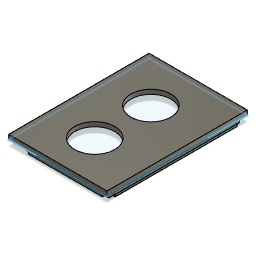
Buttons_Prototype (Autodesk Fusion 360 design; units mm, degrees)
Autodesk Fusion 360 part; units mm, degrees
(part 1 of 2)
sketch "Sketch1" plane through (0, 0, 0) normal (0, 0, 1) x (1, 0, 0)
  line L0 (-0.0637, 4.3306) -> (-17.0637, 4.3306)
  line L1 (-17.0637, 4.3306) -> (-17.0637, 0.3306)
  line L2 (-17.0637, 0.3306) -> (-0.0637, 0.3306)
  line L3 (-0.0637, 0.3306) -> (-0.0637, 4.3306)
  dimension "d1" = 17
  dimension "d13" = 4
  constraint horizontal L0
  constraint perpendicular L0 L1
  constraint horizontal L2
  constraint perpendicular L2 L3
  measures "d1" distance of L0.start L0.end
  measures "d13" distance of L0.start L2.end
extrude "Extrude1" add sketch "Sketch1" along normal blind 30 and the other way blind 30 makes body 1
mirror "Mirror1" about plane through (-0.0637, 0.3306, 0) normal (1, 0, 0) of bodies 1 makes body 2
combine "Combine1" operation add target body 2 tool bodies 1
sketch "Sketch2" plane through (0, 4.3306, 0) normal (0, 1, 0) x (-1, 0, 0)
  line L0 (-16.9363, 30) -> (-16.9363, -30)
  line L1 (-16.9363, -30) -> (17.0637, -30)
  line L2 (17.0637, -30) -> (17.0637, 30)
  line L3 (17.0637, 30) -> (-16.9363, 30)
  line L4 (-8.6363, -1.4) -> (-8.6363, 21)
  line L5 (-8.6363, 21) -> (8.7637, 21)
  line L6 (8.7637, 21) -> (8.7637, -1.4)
  line L7 (8.7637, -1.4) -> (-8.6363, -1.4)
  line L8 (17.0637, 22.0663) -> (-16.9363, 22.0663) construction
  line L9 (-16.3938, 30.8919) -> (16.5213, 30.8919) construction
  line L10 (0.0637, 30.8919) -> (0.0637, -2.5621) construction
  line L11 (-16.9363, 22.0663) -> (-16.9363, 33.4379) construction
  dimension "d43" = 17.4
  dimension "d44" = 22.4
  dimension "d45" = 17
  dimension "d46" = 8.7
  dimension "d47" = 9
  constraint vertical L4
  constraint horizontal L5
  constraint vertical L6
  constraint perpendicular L4 L7
  constraint coincident L2 L8.start
  constraint coincident L0 L8.end
  constraint perpendicular L0 L8
  constraint perpendicular L0 L9
  constraint midpoint L9 L10.start
  constraint perpendicular L9 L10
  constraint perpendicular L9 L11
  measures "d43" distance of L6.end L4.start
  measures "d44" distance of L6.end L5.end
  measures "d45" distance of L10 L11
  measures "d46" distance of L4 L10
  measures "d47" distance of L3 L5
extrude "Extrude2" cut sketch "Sketch2" against normal blind 10 contours L4 L5 L6 L7 bodies 2
sketch "Sketch4" plane through (0, 4.3306, 0) normal (0, 1, 0) x (-1, 0, 0)
  line L0 (-8.6363, 21) -> (8.7637, 21)
  line L1 (8.7637, 21) -> (8.7637, -1.4)
  line L2 (8.7637, -1.4) -> (-8.6363, -1.4)
  line L3 (-8.6363, -1.4) -> (-8.6363, 21)
  line L4 (-16.9363, 30) -> (-16.9363, -30)
  line L5 (-16.9363, -30) -> (17.0637, -30)
  line L6 (17.0637, -30) -> (17.0637, 30)
  line L7 (17.0637, 30) -> (-16.9363, 30)
  circle A0 centre (12.9637, 9.9412) radius 2.8284
  circle A1 centre (0.0637, -5.6) radius 2.8284
  circle A2 centre (-12.8363, 9.7728) radius 3.1
  circle A3 centre (0.0637, 25.2) radius 2.7801
  line L8 (0, 34) -> (-17, 34) construction
  line L9 (0, 34) -> (0, 33)
  line L10 (35.0061, 10.085) -> (-39.8532, 9.5965) construction
  line L11 (0.0637, -16.6918) -> (0.0637, 38.8918) construction
  dimension "d50" = 6.2
  dimension "d52" = 17
  dimension "d54" = 4.2
  dimension "d55" = 4.2
  dimension "d56" = 4.2
  dimension "d57" = 4.2
  dimension "d58" = 11.2
  dimension "d59" = 8.7
  constraint parallel L7 L8
  constraint perpendicular L8 L9
  constraint coincident A0.centre L10
  constraint coincident A2.centre L10
  constraint perpendicular L7 L11
  constraint coincident A1.centre L11
  constraint coincident A3.centre L11
  measures "d50" diameter of A2
  measures "d52" distance of L8.start L8.end
  measures "d54" distance of L3 A2.centre
  measures "d55" distance of L0 A3.centre
  measures "d56" distance of L1 A0.centre
  measures "d57" distance of L2 A1.centre
  measures "d58" distance of L2.end L10
  measures "d59" distance of L3 L11
extrude "Extrude3" cut sketch "Sketch4" against normal blind 1.7 contours A0 | A1 | A2 | A3 bodies 2
ref_plane "WorkPlane1" through (0, 0, 10) normal (0, 0, 1) x (1, 0, 0)
sketch "Sketch5" plane through (0, 0, 10) normal (0, 0, 1) x (1, 0, 0)
  line L0 (8.6363, 2.6306) -> (8.6363, 0.3626)
  line L1 (-8.7637, 0.3626) -> (-8.7637, 2.6306)
  line L2 (-8.7637, 2.6306) -> (-6.4957, 2.6306)
  line L3 (6.3683, 2.6306) -> (8.6363, 2.6306)
  line L4 (16.9363, 4.3306) -> (-17.0637, 4.3306)
  line L5 (-10, 0) -> (-8.8513, 0)
  line L6 (-8.7637, 2.6306) -> (8.6363, 2.6306) construction
  line L7 (-0.0637, -7.9052) -> (-0.0637, 9.0948) construction
  line L8 (16.9363, 4.3306) -> (16.9363, 0.3306)
  line L9 (-8.7637, 2.6306) -> (-6.4957, 2.6306)
  line L10 (-8.7637, 0.3626) -> (-6.4957, 2.6306)
  line L11 (-8.7637, 0.3626) -> (-5.573, 0.3626) construction
  line L12 (8.6363, 0.3626) -> (6.3683, 2.6306)
  line L13 (8.6363, 0.3626) -> (11.8101, 0.3626) construction
  dimension "d64" = 1.7
  dimension "d67" = 17.4
  dimension "d69" = 17
  dimension "d70" = 8.7
  dimension "d72" = 45
  dimension "d73" = 2.268
  dimension "d74" = 2.268
  dimension "d75" = 135
  constraint vertical L0
  constraint coincident L3.start L2
  constraint horizontal L5
  constraint vertical L7
  constraint horizontal L11
  constraint horizontal L13
  constraint perpendicular L0 L3
  constraint perpendicular L1 L6
  measures "d64" distance of L2 L4
  measures "d67" distance of L1.end L0.start
  measures "d69" distance of L7 L8
  measures "d70" distance of L0 L7
  measures "d72" angle of L10 L11
  measures "d73" distance of L0.start L3.start
  measures "d74" distance of L1.end L2.end
  measures "d75" angle of L12 L13
extrude "Extrude4" add sketch "Sketch5" along normal mid plane 10 bodies 2
extrude "Extrude5" add 1 faces at (-5.7304, 1.6639, 30) along direction (0, 0, 1) blind 39 on bodies 2 bodies 2
pattern_linear "R-Pattern1" count 1 spacing 0 along (-1, 0, 0) count 2 spacing 39 along (0, 0, 1) of "Extrude2", "Extrude3", "Extrude4"
extrude "Extrude6" cut 1 faces at (5.603, 1.6639, -30) along direction (0, 0, 1) blind 20 on bodies 2 bodies 2
sketch "Sketch1 (2)" plane through (0, 0, 0) normal (0, 1, 0) x (1, 0, 0) in component "Cap"
  line L0 (29.4953, 10.2833) -> (68.4953, 10.2833)
  line L1 (68.4953, 10.2833) -> (68.4953, -28.7167)
  line L2 (68.4953, -28.7167) -> (29.4953, -28.7167)
  line L3 (29.4953, -28.7167) -> (29.4953, 10.2833)
  dimension "d86" = 39
  dimension "d87" = 39
  constraint horizontal L0
  constraint vertical L1
  constraint horizontal L2
  constraint vertical L3
  measures "d86" distance of L0.start L0.end
  measures "d87" distance of L0.end L1.end
extrude "Extrude1'" add sketch "Sketch1 (2)" along normal blind 3 separate body makes body 3 in component "Cap"
sketch "Sketch2 (2)" plane through (0, 3, 0) normal (0, 1, 0) x (-1, 0, 0) in component "Cap"
  line L0 (-29.4953, 28.7167) -> (-68.4953, 28.7167)
  line L1 (-68.4953, 28.7167) -> (-68.4953, -10.2833)
  line L2 (-68.4953, -10.2833) -> (-29.4953, -10.2833)
  line L3 (-29.4953, -10.2833) -> (-29.4953, 28.7167)
  circle A0 centre (-48.9953, 9.2167) radius 14
  dimension "d90" = 28
  dimension "d114" = 19.5
  dimension "d115" = 19.5
  measures "d90" diameter of A0
  measures "d114" distance of L0 A0.centre
  measures "d115" distance of L1 A0.centre
extrude "Extrude2'" add sketch "Sketch2 (2)" along normal blind 12.9 contours A0 bodies 3 in component "Cap"
sketch "Sketch3" plane through (0, 0, 0) normal (0, -1, 0) x (1, 0, 0) in component "Cap"
  line L0 (-25.1467, 10) -> (-25.1467, -69)
  line L1 (-25.1467, -69) -> (-17.1467, -69)
  line L2 (-17.1467, -69) -> (-17.1467, 10)
  line L3 (68.4953, 28.7167) -> (29.4953, 28.7167)
  line L4 (29.4953, 28.7167) -> (29.4953, -10.2833)
  line L5 (29.4953, -10.2833) -> (68.4953, -10.2833)
  line L6 (68.4953, -10.2833) -> (68.4953, 28.7167)
  line L7 (48.9953, 40) -> (48.9953, -35.8515) construction
  line L8 (108.8863, 9.2167) -> (25.1963, 9.2167) construction
  line L9 (40.2953, 20.4167) -> (57.6953, 20.4167)
  line L10 (57.6953, 20.4167) -> (57.6953, -1.9833)
  line L11 (57.6953, -1.9833) -> (40.2953, -1.9833)
  line L12 (40.2953, -1.9833) -> (40.2953, 20.4167)
  circle A0 centre (36.0953, 9.2167) radius 3.1
  circle A1 centre (48.9953, 24.6167) radius 3.1
  circle A2 centre (61.8953, 9.2167) radius 3.1
  circle A3 centre (48.9953, -6.1833) radius 3.1
  dimension "d365" = 19.5
  dimension "d367" = 19.5
  dimension "d368" = 17.4
  dimension "d369" = 22.4
  dimension "d370" = 11.2
  dimension "d371" = 8.7
  dimension "d372" = 6.2
  dimension "d373" = 4.2
  dimension "d374" = 4.2
  dimension "d375" = 4.2
  dimension "d376" = 4.2
  constraint perpendicular L5 L7
  constraint perpendicular L6 L8
  constraint horizontal L9
  constraint vertical L10
  constraint horizontal L11
  constraint vertical L12
  constraint coincident L7 A1.centre
  constraint coincident L8 A2.centre
  constraint coincident L7 A3.centre
  constraint equal A1 A3
  constraint equal A2 A3
  constraint equal A0 A3
  constraint coincident L8 A0.centre
  measures "d365" distance of L3 L8
  measures "d367" distance of L6 L7
  measures "d368" distance of L9.start L9.end
  measures "d369" distance of L9.end L10.end
  measures "d370" distance of L8 L9
  measures "d371" distance of L7 L10
  measures "d372" diameter of A3
  measures "d373" distance of L12 A0.centre
  measures "d374" distance of L9 A1.centre
  measures "d375" distance of L11 A3.centre
  measures "d376" distance of L10 A2.centre
extrude "Extrude7" [suppressed]
extrude "Extrude3'" cut sketch "Sketch3" against normal blind 1.7 contours A0 | A1 | A2 | A3 bodies 3 in component "Cap"
sketch "Sketch5 (2)" plane through (0, 0, 0) normal (0, -1, 0) x (1, 0, 0) in component "Cap"
  line L0 (68.4953, 28.7167) -> (29.4953, 28.7167)
  line L1 (29.4953, 28.7167) -> (29.4953, -10.2833)
  line L2 (29.4953, -10.2833) -> (68.4953, -10.2833)
  line L3 (68.4953, -10.2833) -> (68.4953, 28.7167)
  line L4 (29.4953, 28.7167) -> (31.4953, 28.7167)
  line L5 (31.4953, 28.7167) -> (31.4953, -10.2833)
  line L6 (31.4953, -10.2833) -> (29.4953, -10.2833)
  line L7 (29.4953, -10.2833) -> (29.4953, 28.7167)
  line L8 (68.4953, -10.2833) -> (68.4953, 28.7167)
  circle A0 centre (48.9953, 24.6167) radius 3.1
  circle A1 centre (61.8953, 9.2167) radius 3.1
  circle A2 centre (36.0953, 9.2167) radius 3.1
  circle A3 centre (48.9953, -6.1833) radius 3.1
  line L9 (68.4953, 28.7167) -> (66.4953, 28.7167)
  line L10 (66.4953, 28.7167) -> (66.4953, -10.2833)
  line L11 (66.4953, -10.2833) -> (68.4953, -10.2833)
  line L12 (68.4953, -10.2833) -> (68.4953, 28.7167)
  dimension "d110" = 2
  dimension "d377" = 2
  constraint horizontal L4
  constraint vertical L5
  constraint horizontal L6
  constraint vertical L7
  constraint coincident L2 L5.end
  constraint coincident L0.end L1.start
  constraint vertical L8
  constraint coincident L0.start L3.end
  constraint horizontal L9
  constraint vertical L10
  constraint horizontal L11
  constraint vertical L12
  constraint coincident L2 L10.end
  measures "d110" distance of L0.end L4.end
  measures "d377" distance of L0.start L9.end
sketch "Sketch7" plane through (0, 0, 0) normal (0, 0, 1) x (1, 0, 0)
sketch "Sketch8" plane through (0, 4.3306, 0) normal (0, 1, 0) x (-1, 0, 0)
  line L0 (-16.9363, -10) -> (17.0637, -10)
  line L1 (17.0637, -10) -> (17.0637, 69)
  line L2 (17.0637, 69) -> (-16.9363, 69)
  line L3 (-16.9363, 69) -> (-16.9363, -10)
  line L4 (-8.6363, 21) -> (8.7637, 21)
  line L5 (8.7637, 21) -> (8.7637, -1.4)
  line L6 (8.7637, -1.4) -> (-8.6363, -1.4)
  line L7 (-8.6363, -1.4) -> (-8.6363, 21)
  circle A0 centre (12.9637, 9.9412) radius 2.8284
  circle A1 centre (0.0637, -5.6) radius 2.8284
  circle A2 centre (0.0637, 25.2) radius 2.7801
  circle A3 centre (-12.8363, 9.7728) radius 3.1
  line L8 (-8.6363, 60) -> (8.7637, 60)
  line L9 (8.7637, 60) -> (8.7637, 37.6)
  line L10 (8.7637, 37.6) -> (-8.6363, 37.6)
  line L11 (-8.6363, 37.6) -> (-8.6363, 60)
  circle A4 centre (12.9637, 48.9412) radius 2.8284
  circle A5 centre (0.0637, 33.4) radius 2.8284
  circle A6 centre (0.0637, 64.2) radius 2.7801
  circle A7 centre (-12.8363, 48.7728) radius 3.1
sketch "Sketch9" plane through (0, 3.3018, 0) normal (0, 1, 0) x (-1, 0, 0)
  line L0 (-24.8533, -10) -> (-16.8533, -10)
  line L1 (-16.8533, -10) -> (-16.8533, 69)
  line L2 (-16.8533, 69) -> (-24.8533, 69)
  line L3 (-24.8533, 69) -> (-24.8533, -10)
  circle A0 centre (-20.8533, 64) radius 1.4
  circle A1 centre (21.1467, 64) radius 1.4
  line L4 (17.1467, 69) -> (25.1467, 69)
  line L5 (25.1467, -10) -> (25.1467, 69)
  dimension "d116" = 2.8
  dimension "d117" = 5
  dimension "d118" = 5
  dimension "d119" = 4
  dimension "d120" = 4
  constraint equal A0 A1
  measures "d116" diameter of A0
  measures "d117" distance of L2 A0.centre
  measures "d118" distance of A1.centre L4
  measures "d119" distance of A1.centre L5
  measures "d120" distance of L3 A0.centre
extrude "Extrude8" cut sketch "Sketch9" against normal blind 4 contours A0 | A1 bodies 2
sketch "Sketch10" plane through (0, 3.3018, 0) normal (0, 1, 0) x (-1, 0, 0)
  circle A0 centre (-20.8533, 64) radius 1.4
  line L0 (-24.8533, -10) -> (-16.8533, -10)
  line L1 (-16.8533, -10) -> (-16.8533, 69)
  line L2 (-16.8533, 69) -> (-24.8533, 69)
  line L3 (-24.8533, 69) -> (-24.8533, -10)
  circle A1 centre (-20.8533, 64) radius 2.1574
  circle A2 centre (21.1467, 64) radius 2.1574
  circle A3 centre (21.1467, 64) radius 1.4
  dimension "d123" = 4.3148
  constraint concentric A0 A1
  constraint equal A1 A2
  constraint concentric A2 A3
  measures "d123" diameter of A1
extrude "Extrude9" cut sketch "Sketch10" against normal blind 1.2954 contours A1 | A2 bodies 2
pattern_linear "R-Pattern2" count 2 spacing 69 along (0, 0, -1) of "Extrude8", "Extrude9"
sketch "Sketch11" plane through (0, 3.3018, 0) normal (0, 1, 0) x (-1, 0, 0)
  circle A0 centre (-20.8533, -5) radius 2.1574
  circle A1 centre (-20.8533, 64) radius 2.1574
  line L0 (-24.8533, -10) -> (-16.8533, -10)
  line L1 (-16.8533, -10) -> (-16.8533, 69)
  line L2 (-16.8533, 69) -> (-24.8533, 69)
  line L3 (-16.8533, 0) -> (-24.8533, 0)
  line L4 (-24.8533, 0) -> (-24.8533, 59)
  line L5 (-24.8533, 59) -> (-16.8533, 59)
  line L6 (-16.8533, 59) -> (-16.8533, 0)
  line L7 (25.1467, 59) -> (17.1467, 59)
  line L8 (17.1467, 59) -> (17.1467, 0)
  line L9 (17.1467, 0) -> (25.1467, 0)
  line L10 (25.1467, 0) -> (25.1467, 59)
  line L11 (17.1467, 69) -> (25.1467, 69)
  line L12 (17.1467, -10) -> (25.1467, -10)
  line L13 (25.1467, -10) -> (25.1467, 69)
  dimension "d132" = 10
  dimension "d133" = 10
  dimension "d136" = 8
  dimension "d137" = 8
  dimension "d138" = 10
  dimension "d139" = 10
  constraint horizontal L3
  constraint vertical L4
  constraint horizontal L5
  constraint vertical L6
  constraint coincident L1 L3.start
  constraint vertical L8
  constraint horizontal L9
  constraint vertical L10
  constraint collinear L10 L13
  measures "d132" distance of L2 L5
  measures "d133" distance of L0 L3
  measures "d136" distance of L4.end L5.end
  measures "d137" distance of L7.start L7.end
  measures "d138" distance of L7 L11
  measures "d139" distance of L9 L12
extrude "Extrude10" cut sketch "Sketch11" against normal blind 4 contours L1 L3 L4 L5 L6 | L7 L8 L9 L10 L13 bodies 2
sketch "Sketch1 (3)" plane through (0, 0, 0) normal (0, 1, 0) x (1, 0, 0) in component "Cover top"
  circle A0 centre (116.6706, -10) radius 14.5
  line L0 (137.33, -17.9988) -> (133.9274, 3.8922)
  line L1 (133.9274, 3.8922) -> (113.268, 11.8909)
  line L2 (113.268, 11.8909) -> (96.0112, -2.0012)
  line L3 (96.0112, -2.0012) -> (99.4138, -23.8922)
  line L4 (99.4138, -23.8922) -> (120.0732, -31.8909)
  line L5 (120.0732, -31.8909) -> (137.33, -17.9988)
  point P0 (116.6706, -10)
  dimension "d140" = 29
  measures "d140" diameter of A0
extrude "Extrude1''" add sketch "Sketch1 (3)" along normal blind 3 separate body makes body 4 in component "Cover top"
fillet "Fillet1" radius 1 1 edges at (128.7016, 3, 24.9448) on bodies 4 in component "Cover top"
fillet "Fillet2" radius 1 9 edges at (109.2051, 3, 27.6831) (119.7578, 2.7071, 31.7688) (120.0732, 1, 31.8909) (137.33, 1, 17.9988) (137.2781, 2.7071, 17.6646) (135.54, 3, 6.4828) (123.5977, 3, -7.8916) (97.7125, 3, 12.9467) (104.6396, 3, -4.9448) on bodies 4 in component "Cover top"
sketch "Sketch15" plane through (0, 0, 0) normal (0, 1, 0) x (-1, 0, 0)
sketch "Sketch1 (4)" plane through (0, 0, 0) normal (0, 0, 1) x (1, 0, 0) in component "Box"
  line L0 (-116.6556, 53.5174) -> (-46.6556, 53.5174)
  line L1 (-46.6556, 53.5174) -> (-46.6556, -6.4826)
  line L2 (-46.6556, -6.4826) -> (-116.6556, -6.4826)
  line L3 (-116.6556, -6.4826) -> (-116.6556, 53.5174)
  dimension "d149" = 70
  dimension "d150" = 60
  constraint horizontal L0
  constraint vertical L1
  constraint horizontal L2
  constraint vertical L3
  measures "d149" distance of L0.start L0.end
  measures "d150" distance of L0.start L2.end
extrude "Extrude1'''" add sketch "Sketch1 (4)" along normal blind 50 and the other way blind 50 separate body makes body 5 in component "Box"
sketch "Sketch2 (3)" plane through (-93.9993, 53.5174, 74.8295) normal (0, 1, 0) x (-1, 0, 0) in component "Box"
  line L0 (22.6563, -124.8295) -> (22.6563, -24.8295)
  line L1 (22.6563, -24.8295) -> (-47.3437, -24.8295)
  line L2 (-47.3437, -24.8295) -> (-47.3437, -124.8295)
  line L3 (-47.3437, -124.8295) -> (22.6563, -124.8295)
  line L4 (2.6563, -114.8295) -> (-27.3437, -114.8295)
  line L5 (-27.3437, -114.8295) -> (-27.3437, -34.8295)
  line L6 (-27.3437, -34.8295) -> (2.6563, -34.8295)
  line L7 (2.6563, -34.8295) -> (2.6563, -114.8295)
  line L8 (-11.4915, -124.8295) -> (-11.4915, -24.8295) construction
  dimension "d155" = 20
  dimension "d156" = 20
  dimension "d157" = 10
  dimension "d158" = 10
  constraint horizontal L4
  constraint vertical L5
  constraint horizontal L6
  constraint vertical L7
  constraint coincident L3 L8.start
  constraint coincident L1 L8.end
  constraint perpendicular L1 L8
  measures "d155" distance of L0 L7
  measures "d156" distance of L2 L5
  measures "d157" distance of L3 L4
  measures "d158" distance of L1 L6
sketch "Sketch4 (2)" plane through (0, 53.5174, 0) normal (0, 1, 0) x (-1, 0, 0) in component "Box"
  line L0 (66.6556, -40) -> (66.6556, 40)
  line L1 (66.6556, 40) -> (96.6556, 40)
  line L2 (96.6556, 40) -> (96.6556, -40)
  line L3 (96.6556, -40) -> (66.6556, -40)
  line L4 (116.6556, -50) -> (116.6556, 50)
  line L5 (116.6556, 50) -> (46.6556, 50)
  line L6 (46.6556, -50) -> (116.6556, -50)
  line L7 (113.6556, -47) -> (49.6556, -47)
  line L8 (49.6556, 47) -> (113.6556, 47)
  line L9 (113.6556, 47) -> (113.6556, -47)
  line L10 (116.6556, -50) -> (116.6556, 50)
  line L11 (116.6556, 50) -> (46.6556, 50)
  line L12 (46.6556, 50) -> (46.6556, -50)
  line L13 (46.6556, -50) -> (116.6556, -50)
  line L14 (49.6556, 47) -> (49.6556, 40)
  line L15 (49.6556, 40) -> (49.6556, -47)
  dimension "d167" = 3
  dimension "d170" = 3
  dimension "d171" = 3
  dimension "d260" = 3
  constraint horizontal L7
  constraint horizontal L8
  constraint vertical L9
  constraint perpendicular L8 L14
  constraint coincident L7 L15.end
  constraint perpendicular L7 L15
  measures "d167" distance of L4 L9
  measures "d170" distance of L5 L8
  measures "d171" distance of L6 L7
  measures "d260" distance of L12 L15
extrude "Extrude3''" cut sketch "Sketch4 (2)" against normal blind 23 contours L7 L8 L9 L14 L15 bodies 5 in component "Box"
sketch "Sketch6" plane through (0, 0, 0) normal (0, 1, 0) x (1, 0, 0) in component "Box"
sketch "Sketch7 (2)" plane through (0, 30.5174, 0) normal (0, 1, 0) x (-1, 0, 0) in component "Box"
  line L0 (42.6223, -47) -> (98.8748, -47) construction
  line L1 (110.5382, -35) -> (59.6556, -35) construction
  line L2 (53.4031, 35) -> (110.5382, 35) construction
  line L3 (15.5936, 0) -> (180.7808, 0) construction
  line L4 (105.8748, -50) -> (35.8748, -50)
  circle A0 centre (102.6556, -30) radius 1.4
  circle A1 centre (60.6556, -30) radius 1.4
  circle A2 centre (60.6556, 30) radius 1.4
  circle A3 centre (102.6556, 30) radius 1.4
  line L5 (106.6556, -35) -> (56.6556, -35)
  line L6 (56.6556, -35) -> (56.6556, 35)
  line L7 (56.6556, 35) -> (106.6556, 35)
  line L8 (106.6556, 35) -> (106.6556, -35)
  line L9 (124.5176, 0) -> (30.7808, 0) construction
  line L10 (81.6556, 61.2819) -> (81.6556, -48.7181) construction
  line L11 (116.6556, -50) -> (116.6556, 50)
  line L12 (98.6556, -35) -> (64.6556, -35)
  line L13 (64.6556, -35) -> (64.6556, 35) construction
  line L14 (64.6556, 35) -> (98.6556, 35)
  line L15 (98.6556, 35) -> (98.6556, -35) construction
  line L16 (49.6556, -47) -> (113.6556, -47)
  line L17 (113.6556, -47) -> (113.6556, 47)
  line L18 (113.6556, 47) -> (49.6556, 47)
  line L19 (49.6556, 47) -> (49.6556, -47)
  line L20 (96.6556, 40) -> (96.6556, -40)
  line L21 (96.6556, -40) -> (66.6556, -40)
  line L22 (66.6556, -40) -> (66.6556, 40)
  line L23 (66.6556, 40) -> (96.6556, 40)
  dimension "d193" = 70
  dimension "d194" = 50
  dimension "d195" = 35
  dimension "d196" = 2.8
  dimension "d197" = 2.8
  dimension "d198" = 5
  dimension "d199" = 5
  dimension "d215" = 50
  dimension "d216" = 35
  dimension "d217" = 25
  dimension "d218" = 70
  dimension "d219" = 35
  dimension "d220" = 8
  dimension "d221" = 8
  dimension "d222" = 4
  dimension "d223" = 5
  dimension "d224" = 5
  dimension "d225" = 4
  dimension "d226" = 4
  dimension "d227" = 5
  dimension "d228" = 4
  constraint horizontal L1
  constraint horizontal L2
  constraint horizontal L3
  constraint equal A0 A1
  constraint equal A1 A2
  constraint horizontal L5
  constraint vertical L6
  constraint horizontal L7
  constraint vertical L8
  constraint coincident L3 L9.start
  constraint coincident L3 L9.end
  constraint perpendicular L8 L9
  constraint perpendicular L4 L10
  constraint horizontal L12
  constraint vertical L13
  constraint horizontal L14
  constraint vertical L15
  constraint coincident L2 L13.end
  constraint coincident L5 L12.start
  measures "d193" distance of L1.start L2.end
  measures "d194" distance of L3 L4
  measures "d195" distance of L2 L3
  measures "d196" diameter of A3
  measures "d197" diameter of A0
  measures "d198" distance of L2 A2.centre
  measures "d199" distance of L2 A3.centre
  measures "d215" distance of L5.start L5.end
  measures "d216" distance of L10 L11
  measures "d217" distance of L8 L10
  measures "d218" distance of L5.end L6.end
  measures "d219" distance of L3 L5
  measures "d220" distance of L8 L15
  measures "d221" distance of L6 L13
  measures "d222" distance of A1.centre L13
  measures "d223" distance of A1.centre L5
  measures "d224" distance of L1 A0.centre
  measures "d225" distance of A0.centre L8
  measures "d226" distance of A3.centre L15
  measures "d227" distance of A3.centre L7
  measures "d228" distance of A2.centre L13
sketch "Sketch18" plane through (0, 0, 0) normal (0, 1, 0) x (1, 0, 0)
sketch "Sketch1 (5)" plane through (0, 0, 0) normal (0, 1, 0) x (1, 0, 0) in component "Cover"
  line L0 (-40.9344, -0.0564) -> (29.0656, -0.0564)
  line L1 (29.0656, -0.0564) -> (29.0656, -100.0564)
  line L2 (29.0656, -100.0564) -> (-40.9344, -100.0564)
  line L3 (-40.9344, -100.0564) -> (-40.9344, -0.0564)
  dimension "d240" = 70
  dimension "d241" = 100
  constraint horizontal L0
  constraint vertical L1
  constraint horizontal L2
  constraint vertical L3
  measures "d240" distance of L0.start L0.end
  measures "d241" distance of L0.end L1.end
extrude "Extrude1''''" add sketch "Sketch1 (5)" along normal blind 3.175 separate body makes body 6 in component "Cover"
sketch "Sketch2 (4)" plane through (0, 3.175, 0) normal (0, 1, 0) x (-1, 0, 0) in component "Cover"
  line L0 (40.9344, 100.0564) -> (-29.0656, 100.0564)
  line L1 (-29.0656, 100.0564) -> (-29.0656, 0.0564)
  line L2 (-29.0656, 0.0564) -> (40.9344, 0.0564)
  line L3 (40.9344, 0.0564) -> (40.9344, 100.0564)
  line L4 (23.3344, 8.9564) -> (-15.6656, 8.9564)
  line L5 (-15.6656, 8.9564) -> (-15.6656, 87.9564)
  line L6 (-15.6656, 87.9564) -> (23.3344, 87.9564)
  line L7 (23.3344, 87.9564) -> (23.3344, 8.9564)
  line L8 (3.8344, 0.0564) -> (3.8344, 130.0564) construction
  line L9 (-78.285, 47.9564) -> (126.7344, 47.9564) construction
  line L10 (-29.0656, 0.0564) -> (-29.0656, 100.0564) construction
  line L11 (40.9344, 0.0564) -> (-29.0656, 0.0564) construction
  circle A0 centre (3.8344, 28.4564) radius 14.25
  line L12 (21.4134, 8.9564) -> (21.4134, 47.9564) construction
  circle A1 centre (3.8344, 68.4564) radius 14.25
  line L13 (23.3344, 48.9564) -> (-98.2656, 48.9564) construction
  dimension "d247" = 39
  dimension "d248" = 79
  dimension "d249" = 32.9
  dimension "d250" = 47.9
  dimension "d251" = 39
  dimension "d253" = 28.5
  dimension "d254" = 19.5
  dimension "d255" = 39
  dimension "d256" = 19.5
  dimension "d257" = 19.5
  constraint horizontal L4
  constraint vertical L5
  constraint horizontal L6
  constraint vertical L7
  constraint coincident L2 L8.start
  constraint perpendicular L0 L8
  constraint perpendicular L3 L9
  constraint coincident L8 A0.centre
  constraint coincident L4 L12.start
  constraint coincident L9 L12.end
  constraint perpendicular L9 L12
  constraint coincident L8 A1.centre
  constraint equal A0 A1
  constraint coincident L7 L13.start
  constraint perpendicular L7 L13
  measures "d247" distance of L4.start L4.end
  measures "d248" distance of L4.start L6.end
  measures "d249" distance of L8 L10
  measures "d250" distance of L9 L11
  measures "d251" distance of L4 L9
  measures "d253" diameter of A0
  measures "d254" distance of L9 A0.centre
  measures "d255" distance of L6 L13
  measures "d256" distance of L6 A1.centre
  measures "d257" distance of L5 L8
extrude "Extrude2''" cut sketch "Sketch2 (4)" against normal blind 20 contours A0 | A1 bodies 6 in component "Cover"
sketch "Sketch9 (2)" plane through (0, 53.5174, 0) normal (0, 1, 0) x (-1, 0, 0) in component "Box"
  line L0 (49.6556, 47) -> (113.6556, 47)
  line L1 (113.6556, 47) -> (113.6556, -47)
  line L2 (113.6556, -47) -> (49.6556, -47)
  line L3 (46.6556, 50) -> (46.6556, -50)
  line L4 (46.6556, -50) -> (116.6556, -50)
  line L5 (116.6556, -50) -> (116.6556, 50)
  line L6 (116.6556, 50) -> (46.6556, 50)
  line L7 (49.6556, -47) -> (49.6556, 47)
sketch "Sketch10 (2)" plane through (0, 53.5174, 0) normal (0, 1, 0) x (-1, 0, 0) in component "Box"
sketch "Sketch11 (2)" plane through (-81.6556, 53.5174, 0) normal (0, 1, 0) x (-1, 0, 0) in component "Box"
ref_plane "WorkPlane2" through (-81.6556, 23.5174, 30) normal (0, 0, 1) x (1, 0, 0) in component "Box"
sketch "Sketch8 (2)" plane through (0, 0, 50) normal (0, 0, 1) x (1, 0, 0) in component "Box"
  line L0 (-116.6556, -6.4826) -> (-46.6556, -6.4826)
  line L1 (-46.6556, -6.4826) -> (-46.6556, 53.5174)
  line L2 (-46.6556, 53.5174) -> (-116.6556, 53.5174)
  line L3 (-116.6556, 53.5174) -> (-116.6556, -6.4826)
  line L4 (-111.6556, -3.4826) -> (-51.6556, -3.4826)
  line L5 (-51.6556, -3.4826) -> (-51.6556, 21.5174)
  line L6 (-51.6556, 21.5174) -> (-111.6556, 21.5174)
  line L7 (-111.6556, 21.5174) -> (-111.6556, -3.4826)
  dimension "d232" = 60
  dimension "d233" = 3
  dimension "d234" = 25
  dimension "d235" = 5
  constraint horizontal L4
  constraint vertical L5
  constraint horizontal L6
  constraint vertical L7
  measures "d232" distance of L4.start L4.end
  measures "d233" distance of L0 L4
  measures "d234" distance of L4.start L6.end
  measures "d235" distance of L3 L7
extrude "Extrude6'" cut sketch "Sketch8 (2)" along normal blind -5 and the other way blind 95 contours L4 L5 L6 L7 bodies 5 in component "Box"
sketch "Sketch17" plane through (-43.9231, 0, 0) normal (1, 0, 0) x (0, 0, -1)
  line L0 (22.0668, 15.9767) -> (-71.9332, 15.9767)
  line L1 (-71.9332, 15.9767) -> (-71.9332, -7.0233)
  line L2 (-71.9332, -7.0233) -> (22.0668, -7.0233)
  line L3 (22.0668, -7.0233) -> (22.0668, 15.9767)
extrude "Extrude5'" cut sketch "Sketch7 (2)" against normal blind 10 contours A0 | A1 | A2 | A3 bodies 5 in component "Box"
sketch "Sketch14" plane through (0, 0, 50) normal (0, 0, 1) x (1, 0, 0) in component "Box"
  line L0 (-116.6556, -6.4826) -> (-46.6556, -6.4826)
  line L1 (-46.6556, -6.4826) -> (-46.6556, 53.5174)
  line L2 (-46.6556, 53.5174) -> (-116.6556, 53.5174)
  line L3 (-116.6556, 53.5174) -> (-116.6556, -6.4826)
  line L4 (-48.6556, 51.5174) -> (-114.6556, 51.5174)
  line L5 (-114.6556, 51.5174) -> (-114.6556, 49.5174)
  line L6 (-114.6556, 49.5174) -> (-48.6556, 49.5174)
  line L7 (-116.6556, 53.5174) -> (-46.6556, 53.5174)
  line L8 (-48.6556, 51.5174) -> (-48.6556, 49.5174)
  line L9 (-46.6556, 53.5174) -> (-46.6556, -6.4826)
  dimension "d263" = 2
  dimension "d264" = 2
  dimension "d265" = 2
  dimension "d337" = 2
  constraint horizontal L4
  constraint vertical L5
  constraint horizontal L6
  constraint perpendicular L6 L8
  measures "d263" distance of L4 L7
  measures "d264" distance of L4.start L6.end
  measures "d265" distance of L3 L5
  measures "d337" distance of L8 L9
extrude "Extrude8'" cut sketch "Sketch14" against normal blind 3 from surface at -2 contours L4 L5 L6 L8 bodies 5 in component "Box"
sketch "Sketch15 (2)" plane through (-46.6556, 0, 0) normal (1, 0, 0) x (0, 0, 1) in component "Box"
  line L0 (-50, -6.4826) -> (50, -6.4826)
  line L1 (-48, 51.5174) -> (-48, 49.1197)
  line L2 (46, 49.1197) -> (46, 51.5174)
  line L3 (-50, -53.5174) -> (50, -53.5174)
  line L4 (50, -53.5174) -> (50, 6.4826)
  line L5 (50, 6.4826) -> (-50, 6.4826)
  line L6 (-50, 6.4826) -> (-50, -53.5174)
  constraint vertical L1
  constraint vertical L2
sketch "Sketch16" plane through (-46.6556, 0, 0) normal (1, 0, 0) x (0, 0, 1) in component "Box"
  line L0 (48, -51.5174) -> (-48, -51.5174)
  line L1 (-48, -51.5174) -> (-48, -49.5174)
  line L2 (-48, -49.5174) -> (48, -49.5174)
  line L3 (48, -49.5174) -> (48, -51.5174)
  line L4 (-50, -53.5174) -> (50, -53.5174)
  line L5 (-50, 6.4826) -> (-50, -53.5174)
  line L6 (50, -53.5174) -> (50, 6.4826)
  dimension "d274" = 2
  dimension "d275" = 2
  dimension "d276" = 2
  dimension "d280" = 2
  constraint horizontal L0
  constraint vertical L1
  constraint horizontal L2
  constraint vertical L3
  measures "d274" distance of L0 L4
  measures "d275" distance of L1 L5
  measures "d276" distance of L2.end L6
  measures "d280" distance of L0.end L1.end
extrude "Extrude9'" cut sketch "Sketch16" against normal blind 3 from surface at -2 bodies 5 in component "Box"
sketch "Sketch17 (2)" plane through (0, 0, -50) normal (0, 0, -1) x (-1, 0, 0) in component "Box"
  line L0 (46.6556, -6.4826) -> (116.6556, -6.4826)
  line L1 (116.6556, -6.4826) -> (116.6556, 53.5174)
  line L2 (116.6556, 53.5174) -> (46.6556, 53.5174)
  line L3 (46.6556, 53.5174) -> (46.6556, -6.4826)
  line L4 (114.6556, 51.5174) -> (48.6556, 51.5174)
  line L5 (48.6556, 51.5174) -> (48.6556, 49.5174)
  line L6 (48.6556, 49.5174) -> (114.6556, 49.5174)
  line L7 (114.6556, 49.5174) -> (114.6556, 51.5174)
  dimension "d281" = 2
  dimension "d282" = 2
  dimension "d283" = 2
  dimension "d284" = 2
  constraint horizontal L4
  constraint vertical L5
  constraint horizontal L6
  constraint vertical L7
  measures "d281" distance of L4.start L6.end
  measures "d282" distance of L2 L4
  measures "d283" distance of L1 L7
  measures "d284" distance of L3 L5
sketch "Sketch18 (2)" plane through (-116.6556, 0, 0) normal (-1, 0, 0) x (0, 0, 1) in component "Box"
  line L0 (-50, -6.4826) -> (50, -6.4826)
  line L1 (50, -6.4826) -> (50, 53.5174)
  line L2 (50, 53.5174) -> (-50, 53.5174)
  line L3 (-50, 53.5174) -> (-50, -6.4826)
  line L4 (-47, -1.4826) -> (47, -1.4826)
  line L5 (47, -1.4826) -> (47, 53.5174)
  line L6 (47, 53.5174) -> (-47, 53.5174)
  line L7 (-47, 53.5174) -> (-47, -1.4826)
  dimension "d285" = 3
  dimension "d286" = 5
  dimension "d287" = 3
  constraint horizontal L4
  constraint vertical L5
  constraint horizontal L6
  constraint vertical L7
  constraint coincident L2 L5.end
  measures "d285" distance of L1 L5
  measures "d286" distance of L0 L4
  measures "d287" distance of L3 L7
extrude "Extrude10'" cut sketch "Sketch18 (2)" against normal blind 5 contours L2 L4 L5 L6 L7 bodies 5 in component "Box"
sketch "Sketch19" plane through (0, 0, 47) normal (0, 0, -1) x (-1, 0, 0) in component "Box"
  line L0 (114.6556, 49.5174) -> (49.6556, 49.5174)
  line L1 (111.6556, 30.5174) -> (111.6556, -1.4826)
  line L2 (111.6556, -1.4826) -> (116.6556, -1.4826)
  line L3 (116.6556, -1.4826) -> (116.6556, 53.5174)
  line L4 (116.6556, 53.5174) -> (49.6556, 53.5174)
  line L5 (49.6556, 51.5174) -> (114.6556, 51.5174)
  line L6 (114.6556, 51.5174) -> (114.6556, 49.5174)
  line L7 (114.6556, 53.467) -> (112.6556, 53.467)
  line L8 (112.6556, 53.467) -> (112.6556, -1.4826)
  line L9 (112.6556, -1.4826) -> (114.6556, -1.4826)
  line L10 (114.6556, -1.4826) -> (114.6556, 53.467)
  line L11 (116.6556, -6.4826) -> (116.6556, 53.5174)
  line L12 (46.6556, -6.4826) -> (116.6556, -6.4826)
  line L13 (49.6556, 53.5174) -> (49.6556, 51.5174)
  line L14 (49.6556, 49.5174) -> (49.6556, 30.5174)
  line L15 (49.6556, 30.5174) -> (111.6556, 30.5174)
  line L16 (114.6556, 53.467) -> (114.6556, 49)
  dimension "d290" = 2
  dimension "d293" = 5
  dimension "d294" = 2
  constraint vertical L8
  constraint horizontal L9
  constraint vertical L10
  constraint coincident L10 L16.end
  constraint perpendicular L0 L16
  measures "d290" distance of L10 L11
  measures "d293" distance of L9 L12
  measures "d294" distance of L8.end L9.end
extrude "Extrude11" cut sketch "Sketch19" against normal blind 2 contours L0 L2 L8 L9 L10 L16 | L0 L5 L6 L8 L10 L16 | L5 L7 L8 L10 L16 bodies 5 in component "Box"
sketch "Sketch4 (3)" plane through (0, 0, 0) normal (0, 1, 0) x (1, 0, 0) in component "Cover"
  line L0 (20.0656, -96.5564) -> (-38.7344, -96.5564)
  line L1 (-38.7344, -96.5564) -> (-38.7344, -3.5564)
  line L2 (-38.7344, -3.5564) -> (20.0656, -3.5564)
  line L3 (20.0656, -6.5564) -> (-35.7344, -6.5564)
  line L4 (-35.7344, -6.5564) -> (-35.7344, -93.5564)
  line L5 (-35.7344, -93.5564) -> (20.0656, -93.5564)
  line L6 (20.0656, -96.5564) -> (20.0656, -93.5564)
  line L7 (29.0656, -0.0564) -> (29.0656, -100.0564)
  line L8 (29.0656, -100.0564) -> (-40.9344, -100.0564)
  line L9 (-40.9344, -100.0564) -> (-40.9344, -0.0564)
  line L10 (-40.9344, -0.0564) -> (29.0656, -0.0564)
  line L11 (20.0656, -6.5564) -> (20.0656, -3.5564)
  dimension "d308" = 3.5
  dimension "d311" = 3
  dimension "d312" = 3.5
  dimension "d320" = 3
  dimension "d338" = 9
  dimension "d385" = 58.8
  dimension "d386" = 55.8
  dimension "d387" = 9
  constraint horizontal L0
  constraint perpendicular L0 L1
  constraint perpendicular L1 L2
  constraint perpendicular L3 L4
  constraint perpendicular L5 L6
  constraint coincident L5 L6.end
  constraint perpendicular L3 L11
  measures "d308" distance of L0 L8
  measures "d311" distance of L0.start L5.end
  measures "d312" distance of L2 L10
  measures "d320" distance of L1 L4
  measures "d338" distance of L7 L11
  measures "d385" distance of L0.start L0.end
  measures "d386" distance of L4.end L5.end
  measures "d387" distance of L6 L7
extrude "Extrude3'''" add sketch "Sketch4 (3)" against normal blind 4 contours L0 L1 L2 L3 L4 L5 L6 L11 bodies 6 in component "Cover"
sketch "Sketch5 (3)" plane through (0, 0, 96.5564) normal (0, 0, 1) x (1, 0, 0) in component "Cover"
  line L0 (20.0656, 0) -> (-38.7344, 0)
  line L1 (-38.7344, 0) -> (-38.7344, -4)
  line L2 (-38.7344, -4) -> (20.0656, -4)
  line L3 (20.0656, -4) -> (20.0656, 0)
  line L4 (-35.7344, -2.5) -> (17.0656, -2.5)
  line L5 (17.0656, -2.5) -> (17.0656, -4)
  line L6 (17.0656, -4) -> (-35.7344, -4)
  line L7 (-35.7344, -4) -> (-35.7344, -2.5)
  line L8 (29.0656, 0) -> (-40.9344, 0)
  dimension "d321" = 2.5
  dimension "d322" = 1.5
  dimension "d323" = 3
  dimension "d324" = 3
  constraint horizontal L4
  constraint vertical L5
  constraint horizontal L6
  constraint vertical L7
  measures "d321" distance of L4 L8
  measures "d322" distance of L4.end L5.end
  measures "d323" distance of L1 L7
  measures "d324" distance of L3 L5
extrude "Extrude4'" add sketch "Sketch5 (3)" along normal blind 1.5 contours L2 L4 L5 L6 L7 bodies 6 in component "Cover"
sketch "Sketch6 (2)" plane through (0, 0, 3.5564) normal (0, 0, -1) x (-1, 0, 0) in component "Cover"
  line L0 (38.7344, 0) -> (-20.0656, 0)
  line L1 (-20.0656, -4) -> (38.7344, -4)
  line L2 (38.7344, -4) -> (38.7344, 0)
  line L3 (-17.0656, -2.5) -> (35.7344, -2.5)
  line L4 (35.7344, -2.5) -> (35.7344, -4)
  line L5 (35.7344, -4) -> (-17.0656, -4)
  line L6 (-17.0656, -4) -> (-17.0656, -2.5)
  line L7 (40.9344, 0) -> (-29.0656, 0)
  line L8 (-20.0656, 0) -> (-20.0656, -4)
  dimension "d327" = 2.5
  dimension "d328" = 3
  constraint horizontal L3
  constraint vertical L4
  constraint horizontal L5
  constraint vertical L6
  constraint coincident L1 L4.end
  measures "d327" distance of L3 L7
  measures "d328" distance of L2 L4
extrude "Extrude5''" add sketch "Sketch6 (2)" along normal blind 1.5 contours L1 L3 L4 L5 L6 bodies 6 in component "Cover"
sketch "Sketch7 (3)" plane through (-38.7344, 0, 0) normal (-1, 0, 0) x (0, 0, 1) in component "Cover"
  line L0 (96.5564, 0) -> (3.5564, 0)
  line L1 (3.5564, 0) -> (3.5564, -4)
  line L2 (3.5564, -4) -> (96.5564, -4)
  line L3 (96.5564, -4) -> (96.5564, 0)
  line L4 (6.5564, -2.5) -> (93.5564, -2.5)
  line L5 (93.5564, -2.5) -> (93.5564, -4)
  line L6 (93.5564, -4) -> (6.5564, -4)
  line L7 (6.5564, -4) -> (6.5564, -2.5)
  line L8 (100.0564, 0) -> (0.0564, 0)
  dimension "d332" = 2.5
  dimension "d333" = 3
  dimension "d334" = 3
  constraint horizontal L4
  constraint vertical L5
  constraint horizontal L6
  constraint vertical L7
  constraint coincident L2 L5.end
  measures "d332" distance of L4 L8
  measures "d333" distance of L3 L5
  measures "d334" distance of L1 L7
extrude "Extrude6''" add sketch "Sketch7 (3)" along normal blind 1.5 contours L2 L4 L5 L6 L7 bodies 6 in component "Cover"
sketch "Sketch20" plane through (-111.6556, 0, 0) normal (-1, 0, 0) x (0, 0, 1) in component "Box"
  line L0 (45, 21.5174) -> (45, -1.4826)
  line L1 (45, -1.4826) -> (47, -1.4826)
  line L2 (47, -1.4826) -> (47, 30.5174)
  line L3 (47, 30.5174) -> (-47, 30.5174)
  line L4 (-47, 30.5174) -> (-47, -1.4826)
  line L5 (-47, -1.4826) -> (-45, -1.4826)
  line L6 (-45, -1.4826) -> (-45, 21.5174)
  line L7 (-45, 21.5174) -> (45, 21.5174)
sketch "Sketch8 (3)" plane through (0, 0, 0) normal (0, 1, 0) x (1, 0, 0) in component "Cover"
sketch "Sketch21" plane through (-93.9993, 53.5174, 74.8295) normal (0, 1, 0) x (-1, 0, 0) in component "Box"
  line L0 (22.6563, -124.8295) -> (22.6563, -24.8295)
  line L1 (20.6563, -27.8372) -> (18.6563, -27.8372)
  line L2 (18.6563, -27.8372) -> (18.6563, -25.9523)
  line L3 (18.6563, -25.9523) -> (20.6563, -25.9523)
  line L4 (20.6563, -25.9523) -> (20.6563, -27.8372)
  dimension "d344" = 2
  dimension "d345" = 2
  constraint horizontal L1
  constraint vertical L2
  constraint horizontal L3
  constraint vertical L4
  measures "d344" distance of L2.end L3.end
  measures "d345" distance of L0 L4
extrude "Extrude12" cut sketch "Sketch21" against normal blind 1 bodies 5 in component "Box"
sketch "Sketch22" plane through (0, 0, -47) normal (0, 0, 1) x (1, 0, 0) in component "Box"
  line L0 (-111.6556, 30.5174) -> (-49.6556, 30.5174)
  line L1 (-49.6556, 30.5174) -> (-49.6556, 49.5174)
  line L2 (-49.6556, 49.5174) -> (-51.6556, 49.5174)
  line L3 (-51.6556, 49.5174) -> (-51.6556, 51.5174)
  line L4 (-51.6556, 51.5174) -> (-49.6556, 51.5174)
  line L5 (-49.6556, 51.5174) -> (-49.6556, 53.5174)
  line L6 (-49.6556, 53.5174) -> (-116.6556, 53.5174)
  line L7 (-116.6556, 53.5174) -> (-116.6556, -1.4826)
  line L8 (-116.6556, -1.4826) -> (-111.6556, -1.4826)
  line L9 (-111.6556, -1.4826) -> (-111.6556, 30.5174)
  line L10 (-114.6556, -1.4826) -> (-112.6556, -1.4826)
  line L11 (-112.1556, -1.4826) -> (-112.1556, 53.5174)
  line L12 (-112.1556, 53.5174) -> (-114.6556, 53.5174)
  line L13 (-114.6556, 53.5174) -> (-114.6556, -1.4826)
  line L14 (-116.6556, -6.4826) -> (-116.6556, 53.5174)
  dimension "d348" = 2
  dimension "d349" = 2
  constraint vertical L11
  constraint horizontal L12
  constraint vertical L13
  constraint coincident L6 L11.end
  measures "d348" distance of L13 L14
  measures "d349" distance of L10.start L10.end
extrude "Extrude13" cut sketch "Sketch22" against normal blind 2 contours L6 L8 L10 L11 L12 L13 bodies 5 in component "Box"
sketch "Sketch1 (6)" plane through (0, 0, 0) normal (0, 0, 1) x (1, 0, 0) in component "Left"
  line L0 (66.786, 27.9779) -> (162.286, 27.9779)
  line L1 (162.286, 27.9779) -> (162.286, -26.6471)
  line L2 (162.286, -26.6471) -> (66.786, -26.6471)
  line L3 (66.786, -26.6471) -> (66.786, 27.9779)
  dimension "d352" = 95.5
  dimension "d353" = 54.625
  constraint horizontal L0
  constraint vertical L1
  constraint horizontal L2
  constraint vertical L3
  measures "d352" distance of L0.start L0.end
  measures "d353" distance of L0.end L1.end
extrude "Extrude1'''''" add sketch "Sketch1 (6)" along normal blind 1.6 separate body makes body 7 in component "Left"
sketch "Sketch2 (5)" plane through (0, 0, 1.6) normal (0, 0, 1) x (1, 0, 0) in component "Left"
  line L0 (162.286, -26.6471) -> (162.286, 27.9779)
  line L1 (162.286, 27.9779) -> (66.786, 27.9779)
  line L2 (66.786, 27.9779) -> (66.786, -26.6471)
  line L3 (132.036, -23.6471) -> (132.036, -7.1577) construction
  line L4 (132.036, -7.1577) -> (97.036, -7.1577)
  line L5 (132.036, -7.1577) -> (148.5254, -23.6471)
  line L6 (132.036, -7.1577) -> (164.5606, -7.1577) construction
  line L7 (97.036, -7.1577) -> (80.5466, -23.6471)
  line L8 (97.036, -7.1577) -> (132.036, -7.1577)
  line L9 (114.536, -47.8478) -> (114.536, 40) construction
  line L10 (114.536, -23.6471) -> (148.5254, -23.6471)
  line L11 (80.5466, -23.6471) -> (77.1986, -26.9951)
  line L12 (77.1986, -26.9951) -> (151.4429, -26.9951)
  line L13 (148.5254, -23.6471) -> (151.4429, -26.9951)
  dimension "d356" = 35
  dimension "d357" = 45
  dimension "d358" = 135
  dimension "d359" = 47.75
  dimension "d360" = 17.5
  constraint vertical L3
  constraint horizontal L4
  constraint horizontal L6
  constraint horizontal L8
  constraint vertical L9
  constraint horizontal L10
  constraint parallel L7 L11
  constraint parallel L10 L12
  constraint coincident L9 L10.start
  measures "d356" distance of L3.end L4.end
  measures "d357" angle of L5 L6
  measures "d358" angle of L7 L8
  measures "d359" distance of L0 L9
  measures "d360" distance of L3 L9
extrude "Extrude2'''" cut sketch "Sketch2 (5)" against normal blind 10 bodies 7 in component "Left"
move_body "Move1" bodies 7 to x (0, 0, -1) y (0, 1, 0) z (1, 0, 0) at (161.9564, 0, 24.9906) in component "Left"
copy_body "Body->Comp1" bodies 2 removing the originals makes body 8 in component "Base"
sketch "Sketch23" plane through (-172.6203, 53.5174, -16.7779) normal (0, 1, 0) x (-1, 0, 0) in component "Box"
  line L0 (-105.9647, -23.2221) -> (-75.9647, -23.2221)
  line L1 (-75.9647, -23.2221) -> (-75.9647, 56.7779)
  line L2 (-75.9647, 56.7779) -> (-105.9647, 56.7779)
  line L3 (-105.9647, 56.7779) -> (-105.9647, -23.2221)
  line L4 (-75.9647, -23.2221) -> (-105.9647, -23.2221)
  line L5 (-105.9647, -23.2221) -> (-105.9647, 56.7779)
  line L6 (-105.9647, 56.7779) -> (-75.9647, 56.7779)
  line L7 (-75.9647, 56.7779) -> (-75.9647, -23.2221)
  constraint horizontal L4
  constraint vertical L5
  constraint horizontal L6
  constraint vertical L7
  constraint coincident L2.end L3.start
  constraint coincident L0.end L1.start
extrude "Extrude14" cut 1 faces at (-86.6556, 53.5174, 13.3333) along direction (0, -1, 0) blind 50 on bodies 5 bodies 5 in component "Box"
sketch "Sketch24" plane through (0, 0, -47) normal (0, 0, 1) x (1, 0, 0) in component "Box"
  line L0 (-112.1556, 53.5174) -> (-112.1556, -1.4826)
  line L1 (-112.1556, -1.4826) -> (-111.6556, -1.4826)
  line L2 (-111.6556, -1.4826) -> (-111.6556, 30.5174)
  line L3 (-111.6556, 30.5174) -> (-49.6556, 30.5174)
  line L4 (-49.6556, 30.5174) -> (-49.6556, 49.5174)
  line L5 (-49.6556, 49.5174) -> (-51.6556, 49.5174)
  line L6 (-51.6556, 49.5174) -> (-51.6556, 51.5174)
  line L7 (-51.6556, 51.5174) -> (-49.6556, 51.5174)
  line L8 (-49.6556, 51.5174) -> (-49.6556, 53.5174)
  line L9 (-49.6556, 53.5174) -> (-112.1556, 53.5174)
sketch "Sketch25" plane through (0, 0, -50) normal (0, 0, -1) x (-1, 0, 0) in component "Box"
  line L0 (46.6556, -6.4826) -> (116.6556, -6.4826)
  line L1 (116.6556, -6.4826) -> (116.6556, 53.5174)
  line L2 (116.6556, 53.5174) -> (46.6556, 53.5174)
  line L3 (46.6556, 53.5174) -> (46.6556, -6.4826)
sketch "Sketch26" plane through (0, 0, -50) normal (0, 0, -1) x (-1, 0, 0) in component "Box"
  line L0 (46.6556, -6.4826) -> (116.6556, -6.4826)
  line L1 (116.6556, -6.4826) -> (116.6556, 53.5174)
  line L2 (116.6556, 53.5174) -> (46.6556, 53.5174)
  line L3 (46.6556, 53.5174) -> (46.6556, -6.4826)
  line L4 (48, 51.5174) -> (115, 51.5174)
  line L5 (115, 51.5174) -> (115, 49.5174)
  line L6 (115, 49.5174) -> (48, 49.5174)
  line L7 (48, 49.5174) -> (48, 51.5174)
  line L8 (116.6556, 53.5174) -> (46.6556, 53.5174)
  line L9 (46.6556, -6.4826) -> (116.6556, -6.4826)
  line L10 (116.6556, -6.4826) -> (116.6556, 53.5174)
  line L11 (116.6556, 53.5174) -> (46.6556, 53.5174)
  line L12 (46.6556, 53.5174) -> (46.6556, -6.4826)
  dimension "d380" = 2
  dimension "d381" = 2
  constraint horizontal L4
  constraint vertical L5
  constraint horizontal L6
  constraint vertical L7
  measures "d380" distance of L4 L8
  measures "d381" distance of L4.start L6.end
extrude "Extrude15" cut sketch "Sketch17 (2)" against normal blind 3 from surface at -1 contours L4 L5 L6 L7 bodies 5 in component "Box"
sketch "Sketch19 (2)" plane through (42.5244, 0, 0) normal (-1, 0, 0) x (0, 0, 1)
  line L0 (-10.7344, -39.1811) -> (5.755, -22.6917)
  line L1 (5.755, -22.6917) -> (40.755, -22.6917)
  line L2 (40.755, -22.6917) -> (60.2444, -42.1811)
  line L3 (71.005, -42.1811) -> (71.005, 12.4439)
  line L4 (71.005, 12.4439) -> (-24.495, 12.4439)
  line L5 (-24.495, 12.4439) -> (-24.495, -42.1811)
  line L6 (60.2444, -42.1811) -> (71.005, -42.1811)
  line L7 (-13.3485, -42.1811) -> (-10.7344, -39.1811)
  line L8 (-24.495, -42.1811) -> (-13.3485, -42.1811)
sketch "Sketch20 (2)" plane through (0, 0, 39.0855) normal (0, 0, -1) x (-1, 0, 0)
  line L0 (-72.1003, 16.4625) -> (-72.1003, -38.5375)
  line L1 (-72.1003, -38.5375) -> (-70.1003, -38.5375)
  line L2 (-70.1003, -38.5375) -> (-70.1003, 16.4625)
  line L3 (-70.1003, 16.4625) -> (-72.1003, 16.4625)
  line L4 (-72.5069, 12.4625) -> (-70.0397, 12.4625)
  line L5 (-70.0397, 12.4625) -> (-70.0397, 14.4625)
  line L6 (-70.0397, 14.4625) -> (-72.5069, 14.4625)
  line L7 (-72.5069, 14.4625) -> (-72.5069, 12.4625)
  dimension "d388" = 2
  dimension "d389" = 2
  constraint horizontal L4
  constraint vertical L5
  constraint horizontal L6
  constraint vertical L7
  measures "d388" distance of L4.start L6.end
  measures "d389" distance of L3 L6
extrude "Extrude16" cut sketch "Sketch20 (2)" against normal blind 2 draft -2 contours L0 L2 L4 L6 | L0 L4 L6 L7 sketch seen with x (1, 0, 0) y (0, 1, 0) z (0, 0, 1) at (-186.7559, 37.0549, 7.9145) bodies 5 in component "Box"
sketch "Sketch21 (2)" plane through (70.1003, 0, 0) normal (-1, 0, 0) x (0, 0, 1)
  line L0 (39.0855, 16.4625) -> (39.0855, 14.4625)
  line L1 (39.0855, 14.4625) -> (39.0855, 12.4625)
  line L2 (39.0855, 12.4625) -> (39.0855, -38.5375)
  line L3 (39.0855, -38.5375) -> (-54.9145, -38.5375)
  line L4 (-54.9145, -38.5375) -> (-54.9145, 16.4625)
  line L5 (-54.9145, 16.4625) -> (-57.9145, 16.4625)
  line L6 (-57.9145, 16.4625) -> (-57.9145, -43.5375)
  line L7 (-57.9145, -43.5375) -> (42.0855, -43.5375)
  line L8 (42.0855, -43.5375) -> (42.0855, 16.4625)
  line L9 (42.0855, 16.4625) -> (39.0855, 16.4625)
sketch "Sketch16 (2)" plane through (0, 0, 61.5673) normal (0, 0, 1) x (1, 0, 0)
  line L0 (-34.5696, -27.0546) -> (35.4304, -27.0546)
  line L1 (35.4304, -27.0546) -> (35.4304, 22.9454)
  line L2 (35.4304, 22.9454) -> (-34.5696, 22.9454)
  line L3 (-34.5696, 22.9454) -> (-34.5696, -27.0546)
  line L4 (-14, 26) -> (-14, 22.825)
  line L5 (-14, 22.825) -> (-14, 18)
  dimension "d229" = 3.175
  dimension "d230" = 4.825
  constraint perpendicular L2 L4
  constraint perpendicular L2 L5
  measures "d229" distance of L4.start L4.end
  measures "d230" distance of L4.end L5.end
component "Cap" placed x (1, 0, 0) y (0, 1, 0) z (0, 0, 1) at (33.2922, 69.2358, 163.5794)
component "Cap" placed x (1, 0, 0) y (0, 1, 0) z (0, 0, 1) at (-20.39, 34.65, 60.4884)
component "Cover top" placed x (1, 0, 0) y (0, 1, 0) z (0, 0, 1) at (0.6462, -16.8308, -48.6644)
component "Box" placed x (1, 0, 0) y (0, 1, 0) z (0, 0, 1) at (186.7559, -37.0549, -7.9145)
component "Cover" placed x (-1, 0, 0) y (0, 1, 0) z (0, 0, -1) at (69.39, 15.8189, 72.5614)
component "Left" placed x (1, 0, 0) y (0, 1, 0) z (0, 0, 1) at (-118.8889, -12.534, 112.5573)
component "Base" placed x (1, 0, 0) y (0, 1, 0) z (0, 0, 1) at (0, 0, 0)
component "Cover top" placed x (1, 0, 0) y (0, 1, 0) z (0, 0, 1) at (0.6462, -16.8308, 21.3356)
equation "capL = 22.5 mm"
equation "baseWidth = 37 mm"
equation "baseHeight = 5 mm"
equation "capsenseWidth = 17.4 mm"
equation "capsenseLength = 22.4 mm"
equation "capsenseBase_length = capsenseLength + 3 mm"
equation "capsenseBase_width = 34 mm"
equation "screwHoleID = 2.8 mm"
equation "screwHole_OD = 4.3148 mm"
equation "acrlyic_coverOD = 28 mm"
equation "acrlyicThick = 3.175 mm"
equation "capsenseBase_height = 3 mm"
equation "capsenseThick = 1.5 mm"
equation "coverH = 11 mm"
equation "acrylicCoverOD = 28 mm"
equation "magnL = 5.5 mm"
equation "toleranceFit = 0.2 mm"